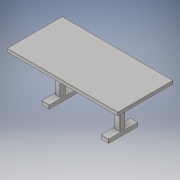
# Autodesk Inventor part: Table
Saved by Autodesk Inventor 2016 (Build 200138000, 138)
## iProperties
Created: 2016-01-30
Part Number: Table
Material: Generic
Document SubType Name: Modeling
Designer: Greg
Density: 1 g/cm^3
Appearance: Default
Author: Greg
Autodesk Inventor part; units mm, degrees
ref_plane "YZ Plane" through (0, 0, 0) normal (1, 0, 0) x (0, 1, 0)
ref_plane "XZ Plane" through (0, 0, 0) normal (0, 1, 0) x (-1, 0, 0)
ref_plane "XY Plane" through (0, 0, 0) normal (0, 0, 1) x (1, 0, 0)
sketch "Sketch1" plane through (0, 0, 0) normal (0, 1, 0) x (-1, 0, 0)
  line L0 (750, -375) -> (-750, -375)
  line L1 (-750, -375) -> (-750, 375)
  line L2 (-750, 375) -> (750, 375)
  line L3 (750, 375) -> (750, -375)
  line L4 (0, 0) -> (-250, 0) construction
  line L5 (0, 0) -> (0, -250) construction
  dimension "d0" = 1500
  dimension "d1" = 750
  dimension "d2" = 250
  dimension "d3" = 250
  constraints: 12 end point, 2 horizontal, 2 parallel, 1 perpendicular, 1 vertical, 2 other
  measures "d0" distance of L1.end L2.end
  measures "d1" distance of L0.end L1.end
  measures "d2" distance of L4.start L4.end
  measures "d3" distance of L4.start L5.end
extrude "Extrusion1" add sketch "Sketch1" along normal blind 40
fillet "Fillet1" radius 10 4 edges at (750, 20, 375) (750, 20, -375) (-750, 20, -375) (-750, 20, 375)
fillet "Fillet2" radius 5 8 edges at (-747.0711, 40, -372.0711) (-750, 40, 0) (-747.0711, 40, 372.0711) (0, 40, 375) (747.0711, 40, 372.0711) (750, 40, 0) (747.0711, 40, -372.0711) (0, 40, -375)
sketch "Sketch2" plane through (0, 0, 0) normal (0, -1, 0) x (1, 0, 0)
  line L0 (0, 0) -> (400, 0) construction
  line L1 (750, -365) -> (750, 365) construction
  line L2 (300, 200) -> (500, 200)
  line L3 (500, 200) -> (500, -200)
  line L4 (500, -200) -> (300, -200)
  line L5 (300, -200) -> (300, 200)
  line L6 (400, 0) -> (400, -100) construction
  line L7 (0, 0) -> (0, 100) construction
  line L8 (-300, 200) -> (-500, 200)
  line L9 (-500, 200) -> (-500, -200)
  line L10 (-500, -200) -> (-300, -200)
  line L11 (-300, -200) -> (-300, 200)
  dimension "d8" = 400
  dimension "d10" = 200
  dimension "d11" = 400
  dimension "d14" = 100
  dimension "d15" = 100
  constraints: 22 end point, 4 symmetric about line, 2 parallel, 2 perpendicular, 2 vertical, 1 horizontal, 2 other
  measures "d8" distance of L0.start L0.end
  measures "d10" distance of L3.end L4.end
  measures "d11" distance of L2.end L3.end
  measures "d14" distance of L0.end L6.end
  measures "d15" distance of L0.start L7.end
extrude "Extrusion2" add sketch "Sketch2" along normal blind 10
sketch "Sketch3" plane through (0, -10, 0) normal (0, -1, 0) x (1, 0, 0)
  line L0 (0, 0) -> (400, 0) construction
  line L1 (400, 0) -> (400, 100) construction
  line L2 (362.5, -37.5) -> (437.5, -37.5)
  line L3 (437.5, -37.5) -> (437.5, 37.5)
  line L4 (437.5, 37.5) -> (362.5, 37.5)
  line L5 (362.5, 37.5) -> (362.5, -37.5)
  line L6 (0, 0) -> (0, 100) construction
  line L7 (-362.5, -37.5) -> (-437.5, -37.5)
  line L8 (-437.5, -37.5) -> (-437.5, 37.5)
  line L9 (-437.5, 37.5) -> (-362.5, 37.5)
  line L10 (-362.5, 37.5) -> (-362.5, -37.5)
  dimension "d18" = 400
  dimension "d19" = 100
  dimension "d20" = 75
  dimension "d21" = 75
  dimension "d22" = 100
  constraints: 22 end point, 4 symmetric about line, 2 horizontal, 2 parallel, 2 vertical, 1 perpendicular, 2 other
  measures "d18" distance of L0.start L0.end
  measures "d19" distance of L0.end L1.end
  measures "d20" distance of L3.end L4.end
  measures "d21" distance of L2.end L3.end
  measures "d22" distance of L0.start L6.end
extrude "Extrusion3" add sketch "Sketch3" along normal blind 500
sketch "Sketch4" plane through (0, -510, 0) normal (0, -1, 0) x (1, 0, 0)
  line L0 (0, 0) -> (400, 0) construction
  line L1 (400, 0) -> (400, 100) construction
  line L2 (400, 0) -> (400, -100) construction
  line L3 (350, 200) -> (450, 200)
  line L4 (450, 200) -> (450, -200)
  line L5 (450, -200) -> (350, -200)
  line L6 (350, -200) -> (350, 200)
  line L7 (0, 0) -> (0, 100) construction
  line L8 (-350, 200) -> (-450, 200)
  line L9 (-450, 200) -> (-450, -200)
  line L10 (-450, -200) -> (-350, -200)
  line L11 (-350, -200) -> (-350, 200)
  dimension "d25" = 400
  dimension "d26" = 100
  dimension "d27" = 100
  dimension "d28" = 100
  dimension "d29" = 400
  dimension "d30" = 100
  constraints: 24 end point, 4 symmetric about line, 3 vertical, 2 horizontal, 2 parallel, 1 perpendicular, 2 other
  measures "d25" distance of L0.start L0.end
  measures "d26" distance of L0.end L1.end
  measures "d27" distance of L0.end L2.end
  measures "d28" distance of L4.end L5.end
  measures "d29" distance of L3.end L4.end
  measures "d30" distance of L0.start L7.end
extrude "Extrusion4" add sketch "Sketch4" along normal blind 50
fillet "Fillet3" radius 5 8 edges at (437.5, -260, -37.5) (362.5, -260, -37.5) (437.5, -260, 37.5) (-362.5, -260, -37.5) (-362.5, -260, 37.5) (-437.5, -260, -37.5) (362.5, -260, 37.5) (-437.5, -260, 37.5)
fillet "Fillet4" radius 5 12 edges at (-400, -510, 200) (-450, -535, 200) (-350, -535, 200) (350, -535, 200) (400, -510, 200) (450, -535, 200) (350, -535, -200) (-450, -535, -200) (-400, -510, -200) (-350, -535, -200) (400, -510, -200) (450, -535, -200)
body "Solid1"
